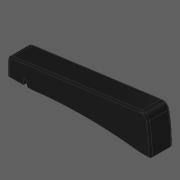
# Autodesk Inventor part: BlackKey0
Saved by Autodesk Inventor 2020 (Build 240168000, 168)
## iProperties
Created: 2019-12-01
Part Number: BlackKey0
Material: PLA Plastic (Black)
Document SubType Name: Modeling
Designer: Isaac Newcomb
Density: 1.06 g/cm^3
Appearance: 3D Printed - Black
Mass: 6.78202 g
Surface Area: 28.9373 cm^2
Volume: 6.39814 cm^3
Project: Ice Keys
hingeDepth: 2.000 mm
edgeSoftenRad: 0.700 mm
slotOffset: 1.174 mm
backWidth: 7.000 mm
hingeRad: 0.500 mm
hingeCutRad: 0.550 mm
slotHeadOffset: 1.000 mm
slotHeadHeight: 3.000 mm
slotHeadWidth: 6.200 mm
neckSlotWidth: 4.300 mm
cutoutWidth: 4.500 mm
keyHeight: 8.000 mm
headHeight: 3.000 mm
headOffset: 1.000 mm
d10: 2.000 mm
blackKeyWidth: 9.600 mm
keySpacing: 0.500 mm
keyLength: 55.000 mm
hingeRadTol: 0.050 mm
hingeRegRadTol: 0.500 mm
Author: Isaac Newcomb
Autodesk Inventor part; units mm, degrees
ref_plane "YZ Plane" through (0, 0, 0) normal (1, 0, 0) x (0, 1, 0)
ref_plane "XZ Plane" through (0, 0, 0) normal (0, 1, 0) x (-1, 0, 0)
ref_plane "Slot Start Plane" through (0, 0, -1.7245) normal (0, 0, 1) x (1, 0, 0)
sketch "Key Profile" plane through (0, 0, 0) normal (1, 0, 0) x (0, 1, 0)
  line L0 (-2, 2.8563) -> (0.684, 1.8794)
  arc A0 (1.6188, -1.1745) -> (0.684, 1.8794) centre (0, 0) ccw
  line L1 (-2, 1.3132) -> (0.1881, 0.5168)
  arc A1 (0, -0.55) -> (0.1881, 0.5168) centre (0, 0) ccw
  line L2 (-2, 2.8563) -> (-2, -0.55)
  line L3 (0, 0) -> (-2, 0) construction
  line L4 (0, -0.55) -> (-2, -0.55)
  line L5 (1.6188, -1.1745) -> (-0.097, -0.55)
  line L6 (6, -5.8029) -> (14, 53.1883)
  line L7 (-2, 54.9636) -> (-2, 2.8563)
  arc A2 (14, 53.1883) -> (-2, 54.9636) centre (0, 0) ccw
  line L8 (-2, -0.55) -> (-2, -7.55)
  arc A3 (4, -7.55) -> (6, -5.8029) centre (4, -5.5317) ccw
  line L9 (-2, -7.55) -> (4, -7.55)
  arc A4 (-2, 2.8563) -> (-2, 50.2011) centre (-188.0444, 26.5287) ccw
  point P0 (-0.5, 26.5287)
  dimension "hingeCutRad" = 0.55
  dimension "hingeDepth" = 2
  dimension "d10" = 2
  dimension "keyLength" = 55
  dimension "blackKeyExtraHeight" = 8
  dimension "keyHeight" = 8
  dimension "d107" = 20
  dimension "d122" = 4
  dimension "slotOffset" = 1.1745
  dimension "backWidth" = 7
  dimension "d129" = 4.7625
  dimension "d130" = 1.5
  constraints: 21 end point, 12 point on circle, 6 tangent, 5 centre point, 4 point on line, 3 coincident, 3 horizontal, 2 parallel, 2 vertical, 1 collinear
  measures "hingeCutRad" radius of A1
  measures "hingeDepth" distance of L3.start L3.end
  measures "d10" radius of A0
  measures "keyLength" radius of A2
  measures "blackKeyExtraHeight" horizontal distance of L6.start L6.end
  measures "keyHeight" distance from line of L6.start L7
  measures "d107" angle of L4 L1
  measures "d122" horizontal distance of A0.centre L9.end
  measures "slotOffset" vertical distance of L5.start point (0, 0)
  measures "backWidth" distance of L2.end L8.end
  measures "d129" distance of L7.start A4.end
  measures "d130" distance from line of L7 point (-0.5, 26.529)
extrude "Key" add sketch "Key Profile" along normal mid plane 9.6 contours A4 L7 A2 L6 A3 L9 L8 L4 L5 A0 L0 | L0 A0 L5 L4 A1 L1 L2
extrude "Protrusion Cutout" cut sketch "Key Profile" along normal mid plane 4.5 contours L0 A0 L5 L4 A1 L1 L2
fillet "Front Fillet" radius 3 1 edges at (0, 14, 53.1883)
sketch "Slot Sketch" plane through (0, 0, -1.7245) normal (0, 0, 1) x (1, 0, 0)
  line L0 (2.15, -2) -> (2.15, 1)
  line L1 (3.1, 4) -> (-3.1, 4)
  line L2 (-2.15, 1) -> (-2.15, -2)
  line L3 (-2.15, -2) -> (2.15, -2)
  line L4 (0, -2) -> (0, 4) construction
  line L5 (-3.1, 4) -> (-3.1, 1)
  line L6 (-3.1, 1) -> (-2.15, 1)
  line L7 (2.15, 1) -> (3.1, 1)
  line L8 (3.1, 1) -> (3.1, 4)
  point P0 (0, 0)
  dimension "d109" = 2
  dimension "slotHeadOffset" = 1
  dimension "slotHeadHeight" = 3
  dimension "slotHeadWidth" = 6.2
  dimension "neckSlotWidth" = 4.3
  constraints: 18 end point, 4 perpendicular, 3 parallel, 2 midpoint, 2 point on line, 2 vertical
  measures "d109" distance from line of point (0, 0) L3
  measures "slotHeadOffset" distance from line of L6 point (0, 0)
  measures "slotHeadHeight" distance of L1.end L5.end
  measures "slotHeadWidth" distance of L1.start L1.end
  measures "neckSlotWidth" distance of L2.end L0.start
extrude "Slot" cut sketch "Slot Sketch" against normal through all
fillet "Edge Softening" radius 0.7 10 edges at (4.8, 13.1123, 52.6256) (4.8, 4.6727, 54.8011) (4.8, 5.3278, -7.0517) (4.8, 1, -7.55) (4.8, 9.8172, 22.3446) (-4.8, 5.3278, -7.0517) (-4.8, 1, -7.55) (-4.8, 13.1123, 52.6256) (-4.8, 4.6727, 54.8011) (-4.8, 9.8172, 22.3446)
equation "\"headHeight\" = 3"
equation "\"headOffset\" = 1"
equation "\"keySpacing\" = 0.5"
equation "\"hingeRadTol\" = 0.05"
equation "\"hingeRegRadTol\" = 0.5"
equation "\"hingeRegWidthTol\" = 0.5"
body "Solid1"
